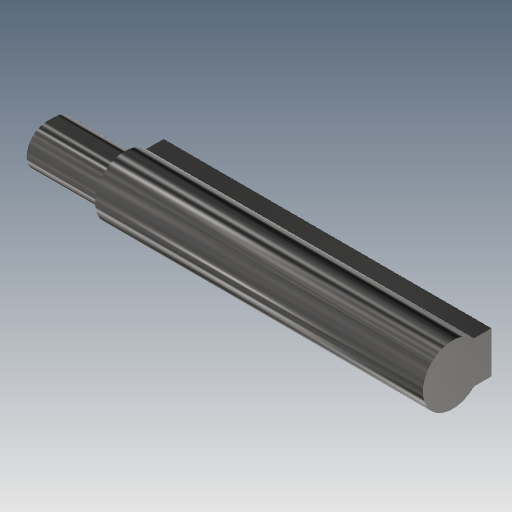
# Autodesk Inventor part: CP96-M9P_SW
Saved by Autodesk Inventor 2021 (Build 250183000, 183)
## iProperties
Part Number: CP96-M9P_SW
Material: Stainless Steel, Polished
Catalog Web Link: www.cadenas.de
Description: CP96 SW-ISO Cylinder:Standard Double Acting,Single/Double Rod
Vendor: SMC
Document SubType Name: Modeling
Designer: partserver
Manufacturer: SMC
Mass: 2.87566 g
Surface Area: 3.98911 cm^2
Volume: 0.359458 cm^3
Density: 8 g/cm^3
Appearance: Stainless - Polished
Category: PARTsolutions
Company: SMC
PSOL_IDENT_0: {$CADENAS_DATA\23d-libs\smc_jp\actuator\standard_air_cylinder\cp96_c96\cp96\parts\cp96_sw.prj},173 {
PSOL_IDENT_1: VTYP=3D},{NB=CP96-M9P_SW},{LINA=CP96-M9P_SW},{NN=CP96 SW},{DATE=18.06.2021 10:30:56},{GEOMDATE=23.04
PSOL_IDENT_2: .2012 00:00:00},{VERSION=},{LINEID=10},{WBVAR=AUTOSWITCH},{WBNUMERIC=}  {NB=CP96-M9P_SW},{LINA=CP96-
PSOL_IDENT_3: M9P_SW},{KT=DUMMY},{AUTOSWITCH=-M9P},{AUTOSWITCHX='','(-) Without autoswitch','-M9N','M9N','-M9P','M
PSOL_IDENT_4: 9P','-M9B','M9B','-M9NW','M9NW','-M9PW','M9PW','-M9BW','M9BW','-M9NA','M9NA','-M9PA','M9PA','-M9BA','
PSOL_IDENT_5: M9BA','-A96','A96','-A93','A93','-A90','A90'},{SWITCH=B}
NB: CP96-M9P_SW
NN: CP96 SW
NT: ISO Cylinder:Standard Double Acting,Single/Double Rod
NBSYN: CP96$AUTOSWITCH._SW
LINA: CP96-M9P_SW
CATALOG: SMC (JP
AUTOSWITCH: M9P Solid state-General-Grommet-Indicator light:Yes-3 wire(PNP)-In line
SUPPLIER: SMC
ARTICLENO: CP96-M9P_SW
BOMINFO: CP96-M9P_SW
CREATOR: CADENAS GmbH
Title: CP96-M9P_SW
Author: Cadenas PARTsolutions
Comments: ISO Cylinder:Standard Double Acting,Single/Double Rod
Autodesk Inventor part; units mm, degrees
sketch "Sketch_12" plane through (0, 0, 0) normal (1, 0, 0) x (0, 1, 0)
  arc A0 (1.4283, 1.4) -> (1.4283, -1.4) centre (0, 0) ccw
  line L0 (1.4283, -1.4) -> (2.6, -1.4)
  line L1 (2.6, -1.4) -> (2.6, 1.4)
  line L2 (2.6, 1.4) -> (1.4283, 1.4)
  constraints: 6 end point, 2 point on circle, 1 centre point
extrude "Extrusion1" add sketch "Sketch_12" along normal blind 22
sketch "Sketch_13" plane through (0, 0, 0) normal (1, 0, 0) x (0, 1, 0)
  line L0 (0.25, 1.35) -> (-0.25, 1.35)
  arc A0 (-0.25, 1.35) -> (-0.25, -1.35) centre (-0.25, 0) ccw
  line L1 (-0.25, -1.35) -> (0.25, -1.35)
  arc A1 (0.25, -1.35) -> (0.25, 1.35) centre (0.25, 0) ccw
  constraints: 4 end point, 4 point on circle, 2 centre point
extrude "Extrusion2" add sketch "Sketch_13" along normal blind 27
sketch "Sketch3" plane through (0, 2.6, 1.4) normal (0, 1, 0) x (1, 0, 0)
  point P0 (2, 1.4)
hole "Hole1" at (2, 2.6, 0) direction (0, -1, 0) diameter 2 depth 0.1
ref_plane "SW_SM_XY" through (0, 0, 0) normal (1, 0, 0) x (0, 0, -1)
ref_plane "SW_SM_YZ" through (0, 0, 0) normal (0, 0, -1) x (0, 1, 0)
ref_plane "SW_SM_ZX" through (0, 0, 0) normal (0, 1, 0) x (1, 0, 0)
body "Solid1"
